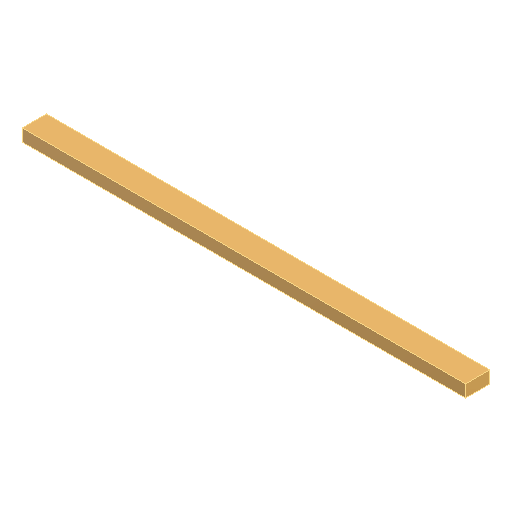
# Autodesk Inventor part: CON-MA08
Saved by Autodesk Inventor 2022 (Build 260153000, 153)
## iProperties
Created: 2022-01-18
Part Number: CON-MA08
Material: Generisch
Document SubType Name: Modeling
Designer: diederichbenedict
Density: 1 g/cm^3
Appearance: MA08, CON-MA08
Author: diederichbenedict
Autodesk Inventor part; units mm, degrees
ref_plane "YZ Plane" through (0, 0, 0) normal (1, 0, 0) x (0, 1, 0)
ref_plane "XZ Plane" through (0, 0, 0) normal (0, 1, 0) x (-1, 0, 0)
ref_plane "XY Plane" through (0, 0, 0) normal (0, 0, 1) x (1, 0, 0)
sketch "MA08, CON-MA08_6" plane through (0, 0, 0) normal (0, 0, 1) x (1, 0, 0)
  line L0 (-9.144, 0.254) -> (9.144, 0.254)
  line L1 (9.144, 0.254) -> (9.144, -0.254)
  line L2 (9.144, -0.254) -> (-9.144, -0.254)
  line L3 (-9.144, -0.254) -> (-9.144, 0.254)
  constraints: 8 end point
extrude "Extrusion1" add sketch "MA08, CON-MA08_6" along normal blind 1
